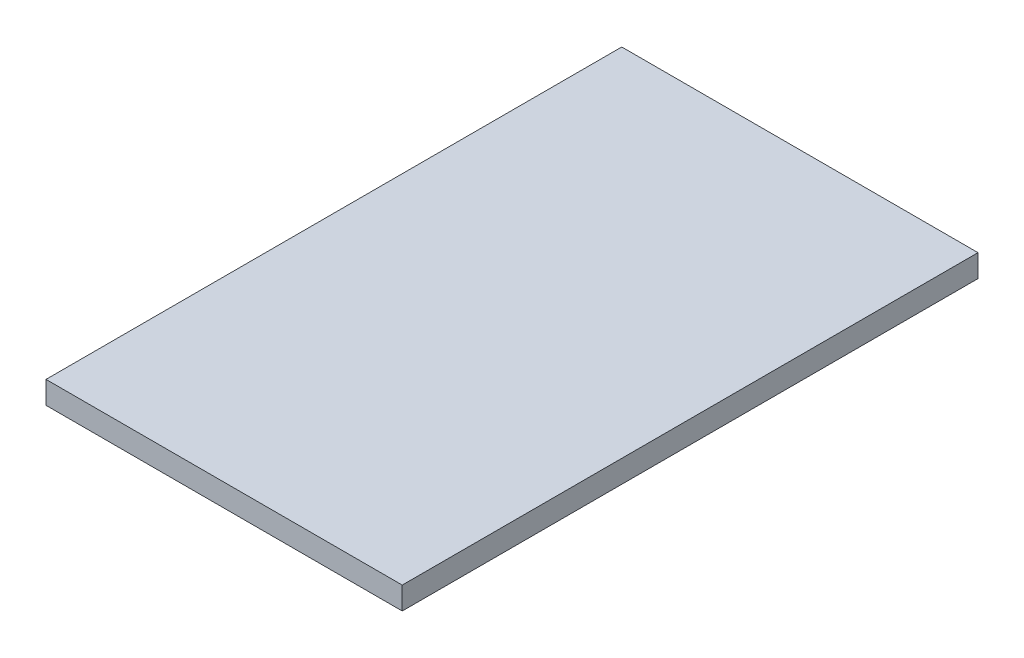
# Autodesk Inventor part: DinMountRelay4
Saved by Autodesk Inventor 2024 (Build 280153000, 153)
## iProperties
Created: 2025-02-14
Part Number: DinMountRelay4
Material: Generic
Document SubType Name: Modeling
Designer: Tommy Rohmann
Density: 1 g/cm^3
Appearance: Default
Author: Tommy Rohmann
Autodesk Inventor part; units mm, degrees
ref_plane "YZ Plane" through (0, 0, 0) normal (1, 0, 0) x (0, 1, 0)
ref_plane "XZ Plane" through (0, 0, 0) normal (0, 1, 0) x (-1, 0, 0)
ref_plane "XY Plane" through (0, 0, 0) normal (0, 0, 1) x (1, 0, 0)
ref_plane "Work Plane1" through (-15.8748, 1.9051, -11.4975) normal (0, 1, 0) x (-1, 0, 0)
sketch "Sketch1" plane through (-15.8748, 1.9051, -11.4975) normal (0, 1, 0) x (-1, 0, 0)
  line L0 (0, 12.7) -> (-46.1627, 12.7) projected
  line L1 (-46.1627, -68.58) -> (0, -68.58) projected
  line L2 (-23.0814, -68.58) -> (-23.0814, 12.7) construction
  line L3 (-23.0814, -68.58) -> (-48.2274, -68.58)
  line L4 (-48.2274, -68.58) -> (-48.2274, 12.7)
  line L5 (-48.2274, 12.7) -> (-23.0814, 12.7)
  line L6 (-48.2274, 9.652) -> (-23.0814, 9.652)
  line L7 (-48.2274, 7.9375) -> (-23.0814, 7.9375)
  line L8 (-48.2274, -65.532) -> (-23.0814, -65.532)
  line L9 (-48.2274, -63.8175) -> (-23.0814, -63.8175)
  line L10 (-46.1627, 12.7) -> (0, 12.7)
  line L11 (0, -68.58) -> (-46.1627, -68.58)
  line L12 (-23.0814, -68.58) -> (2.0646, -68.58)
  line L13 (2.0646, -68.58) -> (2.0646, 12.7)
  line L14 (2.0646, 12.7) -> (-23.0814, 12.7)
  line L15 (2.0646, 9.652) -> (-23.0814, 9.652)
  line L16 (2.0646, 7.9375) -> (-23.0814, 7.9375)
  line L17 (2.0646, -65.532) -> (-23.0814, -65.532)
  line L18 (2.0646, -63.8175) -> (-23.0814, -63.8175)
  point P0 (-15.8748, 11.4975)
  point P1 (0, -68.58)
  dimension "d0" = 25.146
  dimension "d1" = 3.048
  dimension "d2" = 3.048
  dimension "d3" = 4.7625
  dimension "d4" = 4.7625
  constraints: 34 end point, 14 point on line, 10 symmetric about line, 5 perpendicular, 2 midpoint, 1 collinear, 1 horizontal
  measures "d0" distance between parallel lines of L2 L4
  measures "d1" distance between parallel lines of L1 L8
  measures "d2" distance between parallel lines of L0 L6
  measures "d3" distance between parallel lines of L0 L7
  measures "d4" distance between parallel lines of L1 L9
extrude "Extrusion1" add sketch "Sketch1" along normal blind 3.175
body "Solid1"
